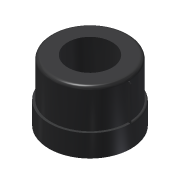
# Autodesk Inventor part: Pipe T with a hole in it
Saved by Autodesk Inventor 2014 SP1 (Build 180222100, 222)
## iProperties
Created: 2014-12-08
Part Number: Pipe T with a hole in it
Material: Generic
Document SubType Name: Modeling
Designer: AlecShufelt
Density: 1 g/cm^3
Appearance: Dark Gray
Author: AlecShufelt
Autodesk Inventor part; units mm, degrees
ref_plane "YZ Plane" through (0, 0, 0) normal (1, 0, 0) x (0, 1, 0)
ref_plane "XZ Plane" through (0, 0, 0) normal (0, 1, 0) x (-1, 0, 0)
ref_plane "XY Plane" through (0, 0, 0) normal (0, 0, 1) x (1, 0, 0)
sketch "Sketch1" plane through (0, 0, 0) normal (0, 1, 0) x (-1, 0, 0)
  circle A0 centre (0, 0) radius 14.732
  dimension "d0" = 29.464
  constraints: 1 centre point, 1 coincident
  measures "d0" diameter of A0
extrude "Extrusion1" add sketch "Sketch1" along normal blind 7.9248
sketch "Sketch2" plane through (0, 7.9248, 0) normal (0, 1, 0) x (1, 0, 0)
  circle A0 centre (0, 0) radius 14.732 projected
  circle A1 centre (0, 0) radius 13.9065
  dimension "d3" = 27.813
  constraints: 1 centre point, 1 coincident
  measures "d3" diameter of A1
extrude "Extrusion2" add sketch "Sketch2" along normal blind 13.97 contours A1
sketch "Sketch4" plane through (0, 7.9248, 0) normal (0, 1, 0) x (1, 0, 0)
  circle A0 centre (0, 0) radius 13.9065 projected
  circle A1 centre (0, 0) radius 14.732 projected
  circle A2 centre (0, 0) radius 13.9065
  circle A3 centre (0, 0) radius 14.732
  line L0 (-13.905, 0.2046) -> (-13.0794, 0.2046) construction
  line L1 (-13.9052, 0.1905) -> (-14.7308, 0.1905)
  line L2 (-13.9052, 0.1905) -> (-13.0796, 0.1905) construction
  line L3 (-13.9052, -0.1905) -> (-14.7308, -0.1905)
  line L4 (-13.9052, -0.1905) -> (-13.0796, -0.1905) construction
  line L5 (-13.9052, 0.1905) -> (14.7308, 0.1896)
  line L6 (-13.9052, -0.1905) -> (14.7307, -0.1927)
  dimension "d7" = 180
  dimension "d8" = 180
  constraints: 14 end point, 9 point on circle, 3 horizontal, 2 centre point, 2 coincident, 2 collinear, 1 concentric, 3 other
  measures "d7" angle of L1 L2
  measures "d8" angle of L3 L4
extrude "Extrusion3" add sketch "Sketch4" along normal blind 12.7 contours L5 A0 L6 | A0 L3 A1 L1 | L5 A1 L6 A0
chamfer "Chamfer1" distance 0.508 angle 45 1 edges at (14.732, 20.6248, 0.0015)
chamfer "Chamfer2" distance 0.508 angle 45 1 edges at (-14.732, 20.6248, 0)
fillet "Fillet1" radius 1.27 1 edges at (-13.9065, 21.8948, 0)
fillet "Fillet2" radius 0.508 1 edges at (0.0004, 7.9248, -14.732)
sketch "Sketch5" plane through (0, 21.8948, 0) normal (0, 1, 0) x (1, 0, 0)
  circle A0 centre (0, 0) radius 12.6365 projected
  circle A1 centre (0, 0) radius 7.9375
  dimension "d19" = 15.875
  constraints: 1 centre point, 1 coincident
  measures "d19" diameter of A1
extrude "Extrusion4" cut sketch "Sketch5" against normal blind 25.4 contours A1
body "Solid1"
